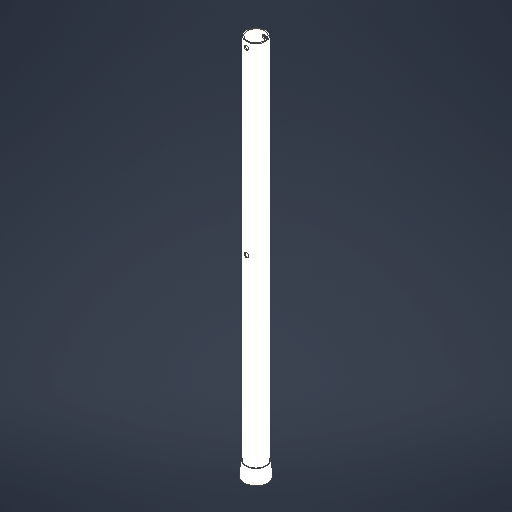
# Autodesk Inventor part: Pieza39
Saved by Autodesk Inventor 2026.2 (Build 302298000, 298)
## iProperties
Created: 2026-01-02
Part Number: Pieza39
Material: Genérico
Document SubType Name: Modeling
Designer: vicho
Density: 1 g/cm^3
Appearance: Valor por defecto
Author: vicho
Autodesk Inventor part; units mm, degrees
ref_plane "YZ Plane" through (0, 0, 0) normal (1, 0, 0) x (0, 1, 0)
sketch "Boceto1" plane through (0, 0, 0) normal (0, 1, 0) x (-1, 0, 0)
  circle A0 centre (0, 0) radius 17.5
  dimension "d0" = 35
  constraints: 1 centre point, 1 coincident
  measures "d0" diameter of A0
extrude "Extrusión1" add sketch "Boceto1" along normal blind 660
shell "Vaciado1" thickness 2 removed faces 2 at (-4.865, 0, -5.1831) at (-4.865, 660, -5.1831)
ref_plane "Plano de trabajo1" through (0, 0, 17.5) normal (0, 0, 1) x (1, 0, 0)
sketch "Boceto2" plane through (0, 0, 17.5) normal (0, 0, 1) x (1, 0, 0)
  line L0 (0, 714.392) -> (0, -104.9263) construction
  line L1 (-367.8002, 0) -> (437.007, 0) construction
  circle A0 centre (0, 650) radius 4
  line L2 (17.5, 660) -> (-17.5, 660) projected
  circle A1 centre (0, 330) radius 4
  point P0 (0, 0)
  dimension "d5" = 8
  dimension "d6" = 10
  dimension "d7" = 8
  dimension "d8" = 330
  constraints: 4 end point, 4 point on line, 2 centre point, 1 horizontal, 1 vertical
  measures "d5" diameter of A0
  measures "d6" distance from line of A0.centre L2
  measures "d7" diameter of A1
  measures "d8" distance from line of L2 A1.centre
extrude "Extrusión2" cut sketch "Boceto2" against normal blind 50
ref_plane "Plano de trabajo2" through (0, 5, 0) normal (0, 1, 0) x (-1, 0, 0)
sketch "Boceto3" plane through (0, 5, 0) normal (0, 1, 0) x (-1, 0, 0)
  circle A0 centre (0, 0) radius 18.5
  dimension "d12" = 37
  constraints: 1 centre point, 1 coincident
  measures "d12" diameter of A0
ref_plane "Plano de trabajo3" through (0, -20, 0) normal (0, 1, 0) x (-1, 0, 0)
sketch "Boceto4" plane through (0, -20, 0) normal (0, 1, 0) x (-1, 0, 0)
  circle A0 centre (0, 0) radius 21
  dimension "d14" = 42
  constraints: 1 centre point, 1 coincident
  measures "d14" diameter of A0
loft "Solevación1" add profiles "Boceto4", "Boceto3"
